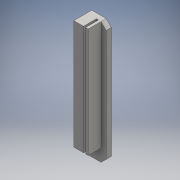
# Autodesk Inventor part: cut platform
Saved by Autodesk Inventor 2016 SP1 (Build 200210100, 210)
## iProperties
Created: 2017-05-09
Part Number: cut platform
Material: Generic
Document SubType Name: Modeling
Designer: Cole
Density: 1 g/cm^3
Appearance: Default
Author: Cole
Autodesk Inventor part; units mm, degrees
ref_plane "YZ Plane" through (0, 0, 0) normal (1, 0, 0) x (0, 1, 0)
ref_plane "XZ Plane" through (0, 0, 0) normal (0, 1, 0) x (-1, 0, 0)
ref_plane "XY Plane" through (0, 0, 0) normal (0, 0, 1) x (1, 0, 0)
sketch "Sketch1" plane through (0, 0, 0) normal (0, 1, 0) x (-1, 0, 0)
  line L0 (45.4816, -24) -> (64.4816, -24)
  line L1 (64.4816, -224) -> (45.4816, -224)
  line L2 (64.4816, -24) -> (52.9072, -24)
  line L3 (45.4816, -51) -> (64.4816, -51)
  line L4 (64.4816, -50.2724) -> (64.4816, -24)
  line L5 (64.4816, -69) -> (45.4816, -69)
  line L6 (45.4816, -51) -> (45.4816, -24)
  line L7 (64.4816, -24) -> (64.4816, -51)
  line L8 (64.4816, -154) -> (45.4816, -154)
  line L9 (64.4816, -204) -> (45.4816, -204)
  line L10 (45.4816, -224) -> (45.4816, -204)
  line L11 (45.4816, -154) -> (45.4816, -69)
  line L12 (64.4816, -69) -> (64.4816, -154)
  line L13 (64.4816, -204) -> (64.4816, -224)
  line L14 (41.4816, -24) -> (36.4816, -24)
  line L15 (36.4816, -24) -> (36.4816, -224)
  line L16 (36.4816, -224) -> (41.4816, -224)
  line L17 (41.4816, -224) -> (41.4816, -24)
  point P0 (0, 0)
  dimension "d0" = 200
  dimension "d1" = 19
  dimension "d7" = 27
  dimension "d9" = 45
  dimension "d11" = 85
  dimension "d12" = 20
  dimension "d13" = 4
  dimension "d14" = 19
  dimension "d15" = 5
  constraints: 36 end point, 13 parallel, 4 perpendicular, 3 horizontal, 2 collinear
  measures "d0" distance of L0.end L1.start
  measures "d1" distance of L1.start L1.end
  measures "d7" distance between parallel lines of L0 L3
  measures "d9" distance between parallel lines of L0 L5
  measures "d11" distance between parallel lines of L8 L5
  measures "d12" distance between parallel lines of L9 L1
  measures "d13" distance between parallel lines of L17 L11
  measures "d14" distance of L8.start L8.end
  measures "d15" distance of L14.start L14.end
extrude "Extrusion2" add sketch "Sketch1" along normal blind 11
sketch "Sketch2" plane through (0, 11, 0) normal (0, 1, 0) x (1, 0, 0)
  line L0 (-64.4816, 224) -> (-36.4816, 224)
  line L1 (-36.4816, 224) -> (-36.4816, 24)
  line L2 (-36.4816, 24) -> (-64.4816, 24)
  line L3 (-64.4816, 24) -> (-64.4816, 224)
  point P0 (0, 0)
  constraints: 8 end point, 2 parallel, 1 horizontal, 1 perpendicular
extrude "Extrusion3" add sketch "Sketch2" along normal blind 3
sketch "Sketch3" plane through (0, 0, 0) normal (0, -1, 0) x (1, 0, 0)
  line L0 (-19.3539, -51.0239) -> (-76.8291, -51.0239)
  line L1 (-76.8291, -51.0239) -> (-76.8291, -110.8451)
  line L2 (-76.8291, -110.8451) -> (-19.3539, -110.8451)
  line L3 (-19.3539, -110.8451) -> (-19.3539, -51.0239)
  line L4 (-25.2187, -135.4773) -> (-86.9948, -135.4773)
  line L5 (-86.9948, -135.4773) -> (-86.9948, -203.9002)
  line L6 (-86.9948, -203.9002) -> (-25.2187, -203.9002)
  line L7 (-25.2187, -203.9002) -> (-25.2187, -135.4773)
  point P0 (0, 0)
  constraints: 16 end point, 4 parallel, 2 horizontal, 2 perpendicular
extrude "Extrusion4" cut sketch "Sketch3" against normal up to surface (11 mm away)
sketch "Sketch4" plane through (0, 14, 0) normal (0, 1, 0) x (1, 0, 0)
  line L0 (-64.4816, 24) -> (-36.4816, 24)
  line L1 (-26.4816, 34) -> (-26.4816, 251)
  line L2 (-36.4816, 261) -> (-64.4816, 261)
  line L3 (-74.4816, 251) -> (-74.4816, 34)
  line L4 (-64.4816, 224) -> (-64.4816, 24) projected
  line L5 (-36.4816, 24) -> (-36.4816, 224) projected
  line L6 (-36.4816, 224) -> (-64.4816, 224) projected
  line L7 (-64.4816, 24) -> (-74.4816, 34)
  line L8 (-36.4816, 24) -> (-26.4816, 34)
  line L9 (-64.4816, 261) -> (-74.4816, 251)
  line L10 (-36.4816, 261) -> (-26.4816, 251)
  point P0 (0, 0)
  point P1 (-74.4816, 24)
  point P2 (-26.4816, 261)
  point P3 (-26.4816, 24)
  point P4 (-74.4816, 261)
  dimension "d22" = 10
  dimension "d23" = 10
  dimension "d24" = 37
  dimension "d31" = 10
  dimension "d32" = 10
  dimension "d33" = 10
  dimension "d34" = 10
  dimension "d35" = 10
  dimension "d36" = 10
  dimension "d37" = 10
  dimension "d38" = 10
  constraints: 16 end point, 8 point on line, 2 parallel, 1 horizontal, 1 perpendicular
  measures "d22" distance between parallel lines of L4 L3
  measures "d23" distance between parallel lines of L1 L5
  measures "d24" distance between parallel lines of L6 L2
  measures "d31" distance of L0.start point (-74.482, 24)
  measures "d32" distance of L3.end point (-74.482, 24)
  measures "d33" distance of L0.end point (-26.482, 24)
  measures "d34" distance of L1.start point (-26.482, 24)
  measures "d35" distance of L2.end point (-74.482, 261)
  measures "d36" distance of L3.start point (-74.482, 261)
  measures "d37" distance of L2.start point (-26.482, 261)
  measures "d38" distance of L1.end point (-26.482, 261)
extrude "Extrusion5" add sketch "Sketch4" along normal blind 21
sketch "Sketch5" plane through (-45.4816, 0, -224) normal (0, 0, -1) x (-1, 0, 0)
  line L0 (-9, 0) -> (-4, 0) projected
  line L1 (-4, 0) -> (-4, 11) projected
  line L2 (0, 11) -> (-4, 11) projected
  line L3 (0, 0) -> (0, 11) projected
  line L4 (19, 0) -> (0, 0) projected
  line L5 (19, 0) -> (19, 14) projected
  line L6 (-9, 14) -> (19, 14) projected
  line L7 (-9, 0) -> (-9, 14) projected
  point P0 (-45.4816, 0)
extrude "Extrusion6" add sketch "Sketch5" along normal blind 13
sketch "Sketch6" plane through (0, 11, 0) normal (0, -1, 0) x (1, 0, 0)
  line L0 (-41.4816, -51.0239) -> (-41.4816, -24) projected
  line L1 (-41.4816, -24) -> (-45.4816, -24) projected
  line L2 (-45.4816, -24) -> (-45.4816, -51) projected
  line L3 (-45.4816, -51) -> (-64.4816, -51) projected
  line L4 (-64.4816, -110.8451) -> (-64.4816, -51) projected
  line L5 (-64.4816, -110.8451) -> (-45.4816, -110.8451) projected
  line L6 (-45.4816, -110.8451) -> (-45.4816, -135.4773) projected
  line L7 (-45.4816, -135.4773) -> (-64.4816, -135.4773) projected
  line L8 (-64.4816, -204) -> (-64.4816, -135.4773) projected
  line L9 (-64.4816, -204) -> (-45.4816, -204) projected
  line L10 (-45.4816, -204) -> (-45.4816, -237) projected
  line L11 (-41.4816, -237) -> (-45.4816, -237) projected
  line L12 (-41.4816, -203.9002) -> (-41.4816, -237) projected
  line L13 (-41.4816, -203.9002) -> (-36.4816, -203.9002) projected
  line L14 (-36.4816, -135.4773) -> (-36.4816, -203.9002) projected
  line L15 (-36.4816, -135.4773) -> (-41.4816, -135.4773) projected
  line L16 (-41.4816, -135.4773) -> (-41.4816, -110.8451) projected
  line L17 (-41.4816, -110.8451) -> (-36.4816, -110.8451) projected
  line L18 (-36.4816, -51.0239) -> (-36.4816, -110.8451) projected
  line L19 (-36.4816, -51.0239) -> (-41.4816, -51.0239) projected
  point P0 (0, 0)
extrude "Extrusion7" cut sketch "Sketch6" against normal up to surface (3 mm away)
sketch "Sketch7" plane through (0, 14, 0) normal (0, -1, 0) x (1, 0, 0)
  line L0 (-36.4816, -110.8451) -> (-36.4816, -135.4773) projected
  line L1 (-41.4816, -135.4773) -> (-36.4816, -135.4773) projected
  line L2 (-41.4816, -110.8451) -> (-41.4816, -135.4773) projected
  line L3 (-36.4816, -110.8451) -> (-41.4816, -110.8451) projected
  line L4 (-41.4816, -51.0239) -> (-36.4816, -51.0239) projected
  line L5 (-41.4816, -24) -> (-41.4816, -51.0239) projected
  line L6 (-45.4816, -24) -> (-41.4816, -24) projected
  line L7 (-45.4816, -51) -> (-45.4816, -24) projected
  line L8 (-64.4816, -51) -> (-45.4816, -51) projected
  line L9 (-64.4816, -51) -> (-64.4816, -24) projected
  line L10 (-64.4816, -24) -> (-74.4816, -34) projected
  line L11 (-74.4816, -34) -> (-74.4816, -251) projected
  line L12 (-74.4816, -251) -> (-64.4816, -261) projected
  line L13 (-64.4816, -261) -> (-36.4816, -261) projected
  line L14 (-36.4816, -261) -> (-26.4816, -251) projected
  line L15 (-26.4816, -251) -> (-26.4816, -34) projected
  line L16 (-26.4816, -34) -> (-36.4816, -24) projected
  line L17 (-36.4816, -24) -> (-36.4816, -51.0239) projected
  line L18 (-36.4816, -203.9002) -> (-36.4816, -237) projected
  line L19 (-36.4816, -237) -> (-41.4816, -237) projected
  line L20 (-41.4816, -203.9002) -> (-41.4816, -237) projected
  line L21 (-36.4816, -203.9002) -> (-41.4816, -203.9002) projected
  line L22 (-45.4816, -110.8451) -> (-64.4816, -110.8451) projected
  line L23 (-45.4816, -135.4773) -> (-45.4816, -110.8451) projected
  line L24 (-64.4816, -135.4773) -> (-45.4816, -135.4773) projected
  line L25 (-64.4816, -135.4773) -> (-64.4816, -110.8451) projected
  line L26 (-45.4816, -204) -> (-64.4816, -204) projected
  line L27 (-45.4816, -237) -> (-45.4816, -204) projected
  line L28 (-45.4816, -237) -> (-64.4816, -237) projected
  line L29 (-64.4816, -237) -> (-64.4816, -204) projected
  point P0 (0, 0)
extrude "Extrusion8" cut sketch "Sketch7" against normal blind 11
sketch "Sketch8" plane through (-64.4816, 0, -204) normal (0, 0, 1) x (1, 0, 0)
  line L0 (0, 0) -> (0, 25) projected
  line L1 (19, 0) -> (0, 0) projected
  line L2 (19, 0) -> (19, 25) projected
  line L3 (19, 25) -> (0, 25) projected
  line L4 (0, 0) -> (0, 25) projected
  line L5 (23, 0) -> (23, 25) projected
  line L6 (28, 0) -> (23, 0) projected
  line L7 (28, 25) -> (28, 0) projected
  line L8 (28, 25) -> (23, 25) projected
  point P0 (64.4816, 0)
extrude "Extrusion9" add sketch "Sketch8" along normal up to surface (180 mm away)
equation "\"d32\" = d31"
equation "\"d33\" = d31"
equation "\"d34\" = d33"
equation "\"d36\" = d35"
equation "\"d38\" = d37"
body "Solid2"
